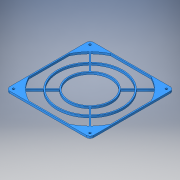
# Autodesk Inventor part: intake2
Saved by Autodesk Inventor 2016 (Build 200138000, 138)
## iProperties
Created: 2015-10-01
Part Number: intake2
Material: Generic
Document SubType Name: Modeling
Designer: xdlea
Density: 1 g/cm^3
Appearance: Cyan
Author: xdlea
Autodesk Inventor part; units mm, degrees
ref_plane "YZ Plane" through (0, 0, 0) normal (1, 0, 0) x (0, 1, 0)
ref_plane "XZ Plane" through (0, 0, 0) normal (0, 1, 0) x (-1, 0, 0)
ref_plane "XY Plane" through (0, 0, 0) normal (0, 0, 1) x (1, 0, 0)
sketch "Sketch1" plane through (0, 0, 0) normal (0, 1, 0) x (-1, 0, 0)
  line L0 (-57.6, 57.6) -> (57.6, 57.6)
  line L1 (57.6, 57.6) -> (57.6, -57.6)
  line L2 (57.6, -57.6) -> (-57.6, -57.6)
  line L3 (-57.6, -57.6) -> (-57.6, 57.6)
  line L4 (-57.6, 57.6) -> (57.6, -57.6) construction
  line L5 (57.6, 57.6) -> (-57.6, -57.6) construction
  circle A0 centre (52.4, 52.4) radius 1.5
  circle A1 centre (52.4, -52.4) radius 1.5
  arc A2 (56.1, 27.5507) -> (27.5507, 56.1) centre (0, 0) ccw
  arc A3 (27.5507, -56.1) -> (56.1, -27.5507) centre (0, 0) ccw
  arc A4 (-56.1, -27.5507) -> (-27.5507, -56.1) centre (0, 0) ccw
  arc A5 (-27.5507, 56.1) -> (-56.1, 27.5507) centre (0, 0) ccw
  line L6 (27.5507, 56.1) -> (-27.5507, 56.1)
  line L7 (-56.1, 27.5507) -> (-56.1, -27.5507)
  line L8 (-27.5507, -56.1) -> (27.5507, -56.1)
  line L9 (56.1, -27.5507) -> (56.1, 27.5507)
  arc A6 (57.6, 52.4) -> (52.4, 57.6) centre (52.4, 52.4) ccw
  line L10 (47.7863, 57.6) -> (44.1942, 44.1942)
  line L11 (44.1942, 44.1942) -> (57.6, 47.7863)
  line L12 (-58, 58) -> (58, 58) construction
  line L13 (58, 58) -> (58, -58) construction
  line L14 (58, -58) -> (-58, -58) construction
  line L15 (-58, -58) -> (-58, 58) construction
  line L16 (-58, 58) -> (58, -58) construction
  line L17 (58, 58) -> (-58, -58) construction
  circle A7 centre (52.4, 52.4) radius 3
  point P0 (0, 56.1)
  dimension "d1" = 3
  dimension "d2" = 104.8
  dimension "d4" = 62.5
  dimension "d9" = 30
  dimension "d80" = 116
  dimension "d81" = 0.4
  dimension "d82" = 1.5
  dimension "d88" = 6
  constraints: 36 end point, 11 point on circle, 8 centre point, 6 equal length, 6 parallel, 6 point on line, 5 coincident, 5 midpoint, 4 equal radius, 3 horizontal, 3 perpendicular, 3 vertical alignment, 2 tangent, 1 horizontal alignment
  measures "d1" diameter of A0
  measures "d2" distance of A1.centre A0.centre
  measures "d4" radius of A2
  measures "d9" angle of L5 L10
  measures "d80" distance of L12.end L13.end
  measures "d81" distance between parallel lines of L1 L13
  measures "d82" distance between parallel lines of L9 L1
  measures "d88" diameter of A7
extrude "Extrusion3" add sketch "Sketch1" along normal blind 2.775 contours L0 L10 L11 L1 L2 L3 | L0 A6 L1 L11 L10 | L0 L1 A6 | A0 | A1 | A7
extrude "Extrusion5" cut sketch "Sketch1" along normal up to next contours L0 L1 A6
sketch "Sketch4" plane through (0, 2.775, 0) normal (0, 1, 0) x (1, 0, 0)
  line L0 (-56.1, -27.5507) -> (-56.1, 27.5507) projected
  arc A0 (-27.5507, 56.1) -> (-56.1, 27.5507) centre (0, 0) ccw projected
  line L1 (-27.5507, 56.1) -> (27.5507, 56.1) projected
  arc A1 (56.1, 27.5507) -> (27.5507, 56.1) centre (0, 0) ccw projected
  line L2 (56.1, 27.5507) -> (56.1, -27.5507) projected
  arc A2 (27.5507, -56.1) -> (56.1, -27.5507) centre (0, 0) ccw projected
  line L3 (27.5507, -56.1) -> (-27.5507, -56.1) projected
  arc A3 (-56.1, -27.5507) -> (-27.5507, -56.1) centre (0, 0) ccw projected
  line L4 (-57.6, 57.6) -> (-57.6, -52.4) projected
  arc A4 (-57.6, -52.4) -> (-52.4, -57.6) centre (-52.4, -52.4) ccw projected
  line L5 (-52.4, -57.6) -> (57.6, -57.6) projected
  line L6 (57.6, -57.6) -> (57.6, 57.6) projected
  line L7 (57.6, 57.6) -> (-57.6, 57.6) projected
  circle A5 centre (0, 0) radius 28
  circle A6 centre (0, 0) radius 29.5
  line L8 (52.4, 52.4) -> (-52.4, -52.4) construction
  line L9 (-21.3832, -20.3226) -> (-44.7213, -43.6607)
  line L10 (-43.6607, -44.7213) -> (-20.3226, -21.3832)
  arc A7 (-52.4, 56.1) -> (-56.1, 52.4) centre (-52.4, 52.4) ccw
  line L11 (-56.1, 52.4) -> (-56.1, -52.4)
  arc A8 (-56.1, -52.4) -> (-52.4, -56.1) centre (-52.4, -52.4) ccw
  line L12 (-52.4, -56.1) -> (52.4, -56.1)
  arc A9 (52.4, -56.1) -> (56.1, -52.4) centre (52.4, -52.4) ccw
  line L13 (56.1, -52.4) -> (56.1, 52.4)
  arc A10 (56.1, 52.4) -> (52.4, 56.1) centre (52.4, 52.4) ccw
  line L14 (52.4, 56.1) -> (-52.4, 56.1)
  arc A11 (-52.4, 55.2) -> (-55.2, 52.4) centre (-52.4, 52.4) ccw
  line L15 (-55.2, 52.4) -> (-55.2, -52.4)
  arc A12 (-55.2, -52.4) -> (-52.4, -55.2) centre (-52.4, -52.4) ccw
  line L16 (-52.4, -55.2) -> (52.4, -55.2)
  arc A13 (52.4, -55.2) -> (55.2, -52.4) centre (52.4, -52.4) ccw
  line L17 (55.2, -52.4) -> (55.2, 52.4)
  arc A14 (55.2, 52.4) -> (52.4, 55.2) centre (52.4, 52.4) ccw
  line L18 (52.4, 55.2) -> (-52.4, 55.2)
  arc A15 (-56.1, -27.5507) -> (-27.5507, -56.1) centre (0, 0) ccw projected
  arc A16 (-55.2, -29.3123) -> (-29.3123, -55.2) centre (0, 0) ccw
  circle A17 centre (0, 0) radius 44.1942 construction
  line L19 (0, 44.1942) -> (44.1942, 44.1942) construction
  circle A18 centre (0, 0) radius 44.9442
  circle A19 centre (0, 0) radius 43.4442
  point P0 (0, 0)
  dimension "d36" = 56
  dimension "d37" = 1.5
  dimension "d38" = 1.5
  dimension "d48" = 0.9
  dimension "d69" = 1.5
  dimension "d70" = 0.75
  constraints: 25 point on circle, 24 end point, 13 centre point, 4 coincident, 3 point on line, 2 parallel, 1 collinear, 1 concentric, 1 horizontal, 1 vertical alignment, 12 other
  measures "d36" diameter of A5
  measures "d37" radial gap between concentric circles of A6 A5
  measures "d38" distance between parallel lines of L9 L10
  measures "d48" distance between parallel lines of L14 L18
  measures "d69" radial gap between concentric circles of A19 A18
extrude "Extrusion12" add sketch "Sketch4" against normal blind 2.775 contours A18 L10 A19 L9 | L9 A19 L10 A18 | A6
extrude "Extrusion13" add sketch "Sketch4" against normal blind 2.775 contours L9 A18 L10 A3 | L9 A19 L10 A18 | L9 A6 L10 A19 picked at (-30.6576, -31.4825) picked at (-23.7298, -24.5548)
extrude "Extrusion15" cut sketch "Sketch1" along normal up to next contours A0
extrude "Extrusion16" cut sketch "Sketch1" along normal blind 1.3875 contours A7
pattern_circular "Circular Pattern8" count 4 over 360 about axis through (0, 2.775, 0) along (0, -1, 0) of "Extrusion15", "Extrusion16", "Extrusion13", "Extrusion5"
equation "\"d1\" = holeSize"
equation "\"d2\" = dHoles"
equation "\"d4\" = 0.5 * fanDia"
equation "\"d82\" = d39"
equation "\"d22\" = thickness"
equation "\"d36\" = fanCenter"
equation "\"d37\" = d39"
equation "\"d38\" = d39"
equation "\"d69\" = d39"
equation "\"d70\" = 0.5 * d39"
equation "\"d62\" = thickness"
equation "\"d64\" = thickness"
equation "\"d89\" = 0.5 * thickness"
equation "\"holeSize\" = 3"
equation "\"thickness\" = 2.775"
equation "\"dHoles\" = 104.8"
equation "\"fanDia\" = 125"
equation "\"d39\" = 1.5"
equation "\"fanCenter\" = 56"
body "Solid1"
